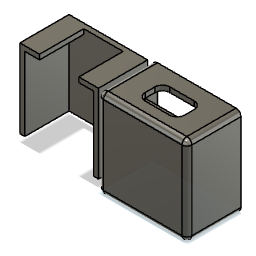
small case v5 (Autodesk Fusion 360 design; units mm, degrees)
Autodesk Fusion 360 part; units mm, degrees
sketch "Esquisse1" plane through (0, 0, 0) normal (0, 0, 1) x (1, 0, 0)
  line L0 (-25, 25) -> (7, 25)
  line L1 (7, 25) -> (7, -7)
  line L2 (7, -7) -> (-25, -7)
  line L3 (-25, -7) -> (-25, 25)
  dimension "d1" = 32
  dimension "d2" = 32
  constraint horizontal L0
  constraint vertical L1
  constraint horizontal L2
  constraint vertical L3
  measures "d1" distance of L0.start L0.end
  measures "d2" distance of L0.end L1.end
extrude "Extrusion1" add sketch "Esquisse1" along normal blind 20 makes body 1
sketch "Esquisse2" plane through (0, 0, 20) normal (0, 0, 1) x (1, 0, 0)
  line L0 (-25, -7) -> (7, -7)
  line L1 (7, -7) -> (7, 25)
  line L2 (7, 25) -> (-25, 25)
  line L3 (-25, 25) -> (-25, -7)
  line L4 (-23, 23) -> (5, 23)
  line L5 (5, 23) -> (5, -7)
  line L6 (5, -7) -> (-23, -7)
  line L7 (-23, -7) -> (-23, 23)
  dimension "d34" = 2
  dimension "d35" = 2
  dimension "d36" = 2
  constraint horizontal L4
  constraint vertical L5
  constraint horizontal L6
  constraint vertical L7
  constraint coincident L0 L5.end
  measures "d34" distance of L3 L7
  measures "d35" distance of L2 L4
  measures "d36" distance of L1 L5
extrude "Extrusion2" cut sketch "Esquisse2" against normal blind 18 contours L0 L4 L5 L6 L7 bodies 1
sketch "Esquisse3" plane through (0, 25, 0) normal (0, 1, 0) x (-1, 0, 0)
  line L0 (-7, 0) -> (25, 0)
  line L1 (25, 0) -> (25, 20)
  line L2 (25, 20) -> (-7, 20)
  line L3 (-7, 20) -> (-7, 0)
  line L4 (17, 2) -> (1, 2)
  line L5 (1, 2) -> (1, 22.0165)
  line L6 (1, 22.0165) -> (17, 22.0165)
  line L7 (17, 22.0165) -> (17, 2)
  dimension "d7" = 8
  dimension "d8" = 8
  dimension "d9" = 2
  constraint horizontal L4
  constraint vertical L5
  constraint horizontal L6
  constraint vertical L7
  measures "d7" distance of L1 L7
  measures "d8" distance of L3 L5
  measures "d9" distance of L0 L4
extrude "Extrusion3" cut sketch "Esquisse3" against normal blind 6 contours L2 L5 L6 L7 | L2 L4 L5 L7 bodies 1
sketch "Esquisse4" plane through (0, 0, 0) normal (0, 0, 1) x (1, 0, 0)
  line L0 (9, 26) -> (45, 26)
  line L1 (45, 26) -> (45, -10)
  line L2 (45, -10) -> (9, -10)
  line L3 (9, -10) -> (9, 26)
  dimension "d13" = 36
  dimension "d14" = 36
  constraint horizontal L0
  constraint vertical L1
  constraint horizontal L2
  constraint vertical L3
  measures "d13" distance of L0.start L0.end
  measures "d14" distance of L0.start L2.end
extrude "Extrusion4" add sketch "Esquisse4" along normal blind 22 separate body makes body 2
sketch "Esquisse5" plane through (0, 26, 0) normal (0, 1, 0) x (-1, 0, 0)
  line L0 (-45, 0) -> (-9, 0)
  line L1 (-9, 0) -> (-9, 22)
  line L2 (-9, 22) -> (-45, 22)
  line L3 (-45, 22) -> (-45, 0)
  line L4 (-22, 6) -> (-32, 6)
  line L5 (-35, 9) -> (-35, 13)
  line L6 (-32, 16) -> (-22, 16)
  line L7 (-19, 13) -> (-19, 9)
  arc A0 (-22, 6) -> (-19, 9) centre (-22, 9) ccw
  arc A1 (-35, 9) -> (-32, 6) centre (-32, 9) ccw
  arc A2 (-32, 16) -> (-35, 13) centre (-32, 13) ccw
  arc A3 (-19, 13) -> (-22, 16) centre (-22, 13) ccw
  dimension "d17" = 10
  dimension "d18" = 10
  dimension "d19" = 6
  dimension "d20" = 6
  dimension "d21" = 3
  constraint horizontal L4
  constraint vertical L5
  constraint horizontal L6
  constraint vertical L7
  constraint tangent L4 A0
  constraint tangent L7 A0
  constraint tangent L4 A1
  constraint tangent L5 A1
  constraint equal A0 A1
  constraint tangent L5 A2
  constraint tangent L6 A2
  constraint equal A0 A2
  constraint tangent L6 A3
  constraint tangent L7 A3
  constraint equal A0 A3
  measures "d17" distance of L1 L7
  measures "d18" distance of L3 L5
  measures "d19" distance of L0 L4
  measures "d20" distance of L2 L6
  measures "d21" radius of A0
extrude "Extrusion5" cut sketch "Esquisse5" against normal blind 4 contours L4 L5 L6 L7 A0 A1 A2 A3 bodies 2
sketch "Esquisse6" plane through (0, -10, 0) normal (0, -1, 0) x (1, 0, 0)
  line L0 (9, 0) -> (45, 0)
  line L1 (45, 0) -> (45, 22)
  line L2 (45, 22) -> (9, 22)
  line L3 (9, 22) -> (9, 0)
sketch "Esquisse7" plane through (0, 0, 0) normal (0, 0, -1) x (-1, 0, 0)
  line L0 (-45, -10) -> (-9, -10)
  line L1 (-9, -10) -> (-9, 26)
  line L2 (-9, 26) -> (-45, 26)
  line L3 (-45, 26) -> (-45, -10)
  line L4 (-11, 24) -> (-43, 24)
  line L5 (-43, 24) -> (-43, 18)
  line L6 (-43, 18) -> (-11, 18)
  line L7 (-11, 18) -> (-11, 24)
  dimension "d38" = 2
  dimension "d39" = 2
  constraint horizontal L4
  constraint vertical L5
  constraint horizontal L6
  constraint vertical L7
  measures "d38" distance of L3 L5
  measures "d39" distance of L1 L7
extrude "Extrusion6" cut sketch "Esquisse7" against normal blind 20 contours L4 L5 L6 L7 bodies 2
sketch "Esquisse8" plane through (0, 0, 0) normal (0, 0, -1) x (-1, 0, 0)
  line L0 (-43, 24) -> (-11, 24)
  line L1 (-11, 24) -> (-11, 18)
  line L2 (-11, 18) -> (-43, 18)
  line L3 (-43, 18) -> (-43, 24)
  line L4 (-45, -10) -> (-9, -10)
  line L5 (-9, -10) -> (-9, 26)
  line L6 (-9, 26) -> (-45, 26)
  line L7 (-45, 26) -> (-45, -10)
  line L8 (-11, 18) -> (-43, 18)
  line L9 (-43, 18) -> (-43, -10)
  line L10 (-43, -10) -> (-11, -10)
  line L11 (-11, -10) -> (-11, 18)
  dimension "d37" = 2
  constraint horizontal L8
  constraint vertical L9
  constraint horizontal L10
  constraint vertical L11
  constraint coincident L4 L9.end
  constraint coincident L1.end L2.start
  measures "d37" distance of L7 L9
extrude "Extrusion7" cut sketch "Esquisse8" against normal blind 7 contours L2 L4 L8 L9 L10 L11 bodies 2
fillet "Congé1" radius 2 4 edges at (9, 26, 11) (45, 26, 11) (45, -10, 11) (9, -10, 11) 1 faces at (21, 2, 22) on bodies 2
sketch "Esquisse9" plane through (0, 0, 7) normal (0, 0, -1) x (-1, 0, 0)
  line L0 (-11, -10) -> (-11, 18)
  line L1 (-11, 18) -> (-43, 18)
  line L2 (-43, 18) -> (-43, -10)
  line L3 (-43, -10) -> (-11, -10)
  line L4 (-11, -10) -> (-13.5, -10)
  line L5 (-13.5, -10) -> (-13.5, 18)
  line L6 (-13.5, 18) -> (-11, 18)
  line L7 (-11, 18) -> (-11, -10)
  line L8 (-43, 18) -> (-40.5, 18)
  line L9 (-40.5, 18) -> (-40.5, -10)
  line L10 (-40.5, -10) -> (-43, -10)
  line L11 (-43, -10) -> (-43, 18)
  dimension "d30" = 2.5
  dimension "d31" = 2.5
  constraint horizontal L4
  constraint vertical L5
  constraint horizontal L6
  constraint vertical L7
  constraint coincident L1 L5.end
  constraint coincident L0.start L3.end
  constraint horizontal L8
  constraint vertical L9
  constraint horizontal L10
  constraint vertical L11
  constraint coincident L3 L9.end
  constraint coincident L1.end L2.start
  measures "d30" distance of L0.start L4.end
  measures "d31" distance of L9.end L2.end
extrude "Extrusion8" cut sketch "Esquisse9" against normal blind 13 contours L0 L1 L3 L4 L5 L6 L7 | L1 L2 L3 L8 L9 L10 L11 bodies 2
sketch "Esquisse10" plane through (27, -10, 11) normal (0, -1, 0) x (1, 0, 0)
  line L0 (15.454, -4) -> (-15, -4)
  line L1 (-15, -4) -> (-15, 9)
  line L2 (-15, 9) -> (15.454, 9)
  line L3 (15.454, 9) -> (15.454, -4)
  constraint horizontal L0
  constraint vertical L1
  constraint horizontal L2
  constraint vertical L3
extrude "Extrusion9" cut sketch "Esquisse10" against normal blind 4 bodies 2
